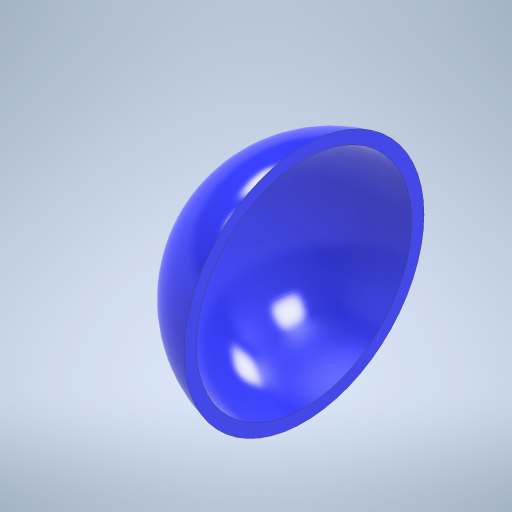
# Autodesk Inventor part: Cabeza R2D2
Saved by Autodesk Inventor 2023 (Build 270158000, 158)
## iProperties
Created: 2022-10-10
Part Number: Cabeza R2D2
Material: Generic
Document SubType Name: Modeling
Designer: User
Density: 1 g/cm^3
Appearance: Default
Author: User
Autodesk Inventor part; units mm, degrees
ref_plane "YZ Plane" through (0, 0, 0) normal (1, 0, 0) x (0, 1, 0)
ref_plane "XZ Plane" through (0, 0, 0) normal (0, 1, 0) x (-1, 0, 0)
ref_plane "XY Plane" through (0, 0, 0) normal (0, 0, 1) x (1, 0, 0)
sketch "Sketch1" plane through (0, 0, 0) normal (0, 1, 0) x (-1, 0, 0)
  line L0 (0, 0) -> (80, 0)
  line L1 (0, 0) -> (0, -100)
  line L2 (0, 0) -> (174.502, 0) construction
  arc A0 (0, -100) -> (80, 0) centre (-22.4371, -0.0503) ccw
  dimension "d0" = 80
  dimension "d1" = 100
  dimension "d5" = 102.4371
  constraints: 6 end point, 2 point on circle, 1 centre point, 1 horizontal, 1 point on line, 1 vertical
  measures "d0" distance of L0.start L0.end
  measures "d1" distance of L0.start L1.end
  measures "d5" radius of A0
revolve "Revolution1" add sketch "Sketch1" angle 360 about axis through (0, 0, 0) along (-1, 0, 0)
shell "Shell1" thickness 10 removed faces 1 at (0, -29.3636, -20.1966)
body "Solid1"
